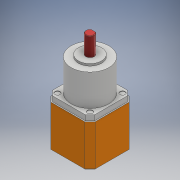
# Autodesk Inventor part: motor con reductora
Saved by Autodesk Inventor 2018 (Build 220112000, 112)
## iProperties
Created: 2019-05-16
Part Number: motor con reductora
Material: Generic
Document SubType Name: Modeling
Designer: JLVega003
Density: 1 g/cm^3
Appearance: Default
Author: JLVega003
Autodesk Inventor part; units mm, degrees
ref_plane "YZ Plane" through (0, 0, 0) normal (1, 0, 0) x (0, 1, 0)
ref_plane "XZ Plane" through (0, 0, 0) normal (0, 1, 0) x (-1, 0, 0)
ref_plane "XY Plane" through (0, 0, 0) normal (0, 0, 1) x (1, 0, 0)
sketch "Sketch1" plane through (0, 0, 0) normal (0, 0, 1) x (1, 0, 0)
  line L0 (-21.15, -21.15) -> (21.15, -21.15)
  line L1 (21.15, -21.15) -> (21.15, 21.15)
  line L2 (21.15, 21.15) -> (-21.15, 21.15)
  line L3 (-21.15, 21.15) -> (-21.15, -21.15)
  line L4 (-21.15, -21.15) -> (21.15, 21.15) construction
  line L5 (21.15, -21.15) -> (-21.15, 21.15) construction
  point P0 (0, 0)
  dimension "d0" = 42.3
  dimension "d1" = 42.3
  constraints: 12 end point, 2 midpoint, 2 parallel, 1 horizontal, 1 perpendicular
  measures "d0" distance of L2.end L1.end
  measures "d1" distance of L1.end L0.end
extrude "Extrusion1" add sketch "Sketch1" along normal blind 40
chamfer "Chamfer1" distance 5 angle 45 4 edges at (21.15, -21.15, 20) (-21.15, -21.15, 20) (21.15, 21.15, 20) (-21.15, 21.15, 20)
sketch "Sketch2" plane through (0, 0, 40) normal (0, 0, 1) x (1, 0, 0)
  circle A0 centre (0, 0) radius 18
  dimension "d7" = 36
  constraints: 1 centre point, 1 coincident
  measures "d7" diameter of A0
extrude "Extrusion2" add sketch "Sketch2" along normal blind 35
sketch "Sketch3" plane through (0, 0, 40) normal (0, 0, 1) x (1, 0, 0)
  circle A0 centre (0, 0) radius 18 projected
  line L0 (-21.15, 16.15) -> (-16.15, 21.15) projected
  line L1 (-21.15, 16.15) -> (-21.15, -16.15) projected
  line L2 (-16.15, -21.15) -> (-21.15, -16.15) projected
  line L3 (-16.15, -21.15) -> (16.15, -21.15) projected
  line L4 (21.15, -16.15) -> (16.15, -21.15) projected
  line L5 (21.15, -16.15) -> (21.15, 16.15) projected
  line L6 (16.15, 21.15) -> (21.15, 16.15) projected
  line L7 (16.15, 21.15) -> (-16.15, 21.15) projected
  line L8 (-15.7358, 20.15) -> (-20.15, 15.7358)
  line L9 (-20.15, 15.7358) -> (-20.15, -15.7358)
  line L10 (-20.15, -15.7358) -> (-15.7358, -20.15)
  line L11 (-15.7358, -20.15) -> (15.7358, -20.15)
  line L12 (15.7358, -20.15) -> (20.15, -15.7358)
  line L13 (20.15, -15.7358) -> (20.15, 15.7358)
  line L14 (20.15, 15.7358) -> (15.7358, 20.15)
  line L15 (15.7358, 20.15) -> (-15.7358, 20.15)
  dimension "d10" = 1
  constraints: 16 end point, 7 other
  measures "d10" distance between parallel lines of L7 L15
extrude "Extrusion3" add sketch "Sketch3" along normal blind 5 contours L15 L14 L13 L12 L11 L10 L9 L8
sketch "Sketch4" plane through (0, 0, 45) normal (0, 0, 1) x (1, 0, 0)
  line L0 (-15.5, -15.5) -> (15.5, -15.5) construction
  line L1 (15.5, -15.5) -> (15.5, 15.5) construction
  line L2 (15.5, 15.5) -> (-15.5, 15.5) construction
  line L3 (-15.5, 15.5) -> (-15.5, -15.5) construction
  line L4 (-15.5, -15.5) -> (15.5, 15.5) construction
  line L5 (15.5, -15.5) -> (-15.5, 15.5) construction
  point P0 (0, 0)
  dimension "d13" = 31
  dimension "d14" = 31
  constraints: 12 end point, 4 coincident, 2 midpoint, 2 parallel, 1 horizontal, 1 perpendicular
  measures "d13" distance of L2.end L1.end
  measures "d14" distance of L1.end L0.end
hole "Hole1" at (-15.5, 15.5, 45) at (15.5, 15.5, 45) at (-15.5, -15.5, 45) at (15.5, -15.5, 45) direction (0, 0, -1) diameter 5 depth 0.5
sketch "Sketch5" plane through (0, 0, 75) normal (0, 0, 1) x (1, 0, 0)
  circle A0 centre (0, 0) radius 11
  dimension "d22" = 22
  constraints: 1 centre point, 1 coincident
  measures "d22" diameter of A0
extrude "Extrusion4" add sketch "Sketch5" along normal blind 2
sketch "Sketch6" plane through (0, 0, 77) normal (0, 0, 1) x (1, 0, 0)
  circle A0 centre (0, 0) radius 4
  dimension "d25" = 8
  constraints: 1 centre point, 1 coincident
  measures "d25" diameter of A0
extrude "Extrusion5" add sketch "Sketch6" along normal blind 18
sketch "Sketch7" plane through (0, 0, 95) normal (0, 0, 1) x (1, 0, 0)
  line L0 (-2.6458, 4) -> (2.6458, 4)
  line L1 (2.6458, 4) -> (2.6458, 3)
  line L2 (2.6458, 3) -> (-2.6458, 3)
  line L3 (-2.6458, 3) -> (-2.6458, 4)
  circle A0 centre (0, 0) radius 4 projected
  line L4 (0, 0) -> (0, 4)
  circle A1 centre (0, 0) radius 4 projected
  point P0 (0, 3)
  dimension "d28" = 7
  constraints: 10 end point, 2 horizontal, 2 parallel, 1 midpoint, 1 perpendicular, 1 point on line, 1 vertical, 1 vertical alignment, 3 other
extrude "Extrusion6" cut sketch "Sketch7" against normal blind 15 contours L0 A0 L3 | L0 L1 A0 | L4 L2 A0 | A0 L2 L4
chamfer "Chamfer2" distance 0.5 angle 45 2 edges at (3.6458, 1.6458, 95) (-1.6458, -3.6458, 95)
chamfer "Chamfer3" distance 1 angle 45 8 edges at (0, 21.15, 0) (18.65, 18.65, 0) (21.15, 0, 0) (-21.15, 0, 0) (-18.65, 18.65, 0) (18.65, -18.65, 0) (0, -21.15, 0) (-18.65, -18.65, 0)
body "Solid1"
